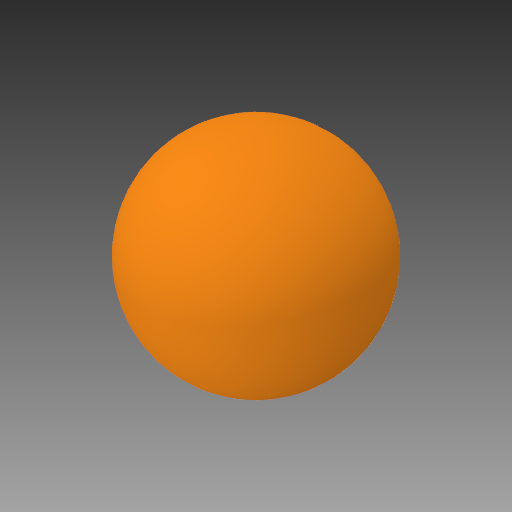
# Autodesk Inventor part: Ball
Saved by Autodesk Inventor 2020 (Build 240168000, 168)
## iProperties
Created: 2019-01-28
Part Number: Ball
Material: Rubber
Document SubType Name: Modeling
Designer: Max Boord
Density: 0.93 g/cm^3
Appearance: Orange
Mass: 796.75 g
Surface Area: 6746.1 cm^2
Volume: 856.72 cm^3
Author: Max Boord
Autodesk Inventor part; units mm, degrees
ref_plane "YZ Plane" through (0, 0, 0) normal (1, 0, 0) x (0, 1, 0)
ref_plane "XZ Plane" through (0, 0, 0) normal (0, 1, 0) x (-1, 0, 0)
ref_plane "XY Plane" through (0, 0, 0) normal (0, 0, 1) x (1, 0, 0)
sketch "Sketch1" plane through (0, 0, 0) normal (0, 1, 0) x (-1, 0, 0)
  circle A0 centre (0, 0) radius 165.1
  dimension "d0" = 330.2
  constraints: 1 centre point, 1 coincident
  measures "d0" diameter of A0
extrude "Extrusion1" add sketch "Sketch1" along normal mid plane 330.2
fillet "Fillet1" radius 165.1 2 edges at (165.1, 165.1, 0) (165.1, -165.1, 0)
shell "Shell1" thickness 2.54 removed faces 0
body "Solid1"
